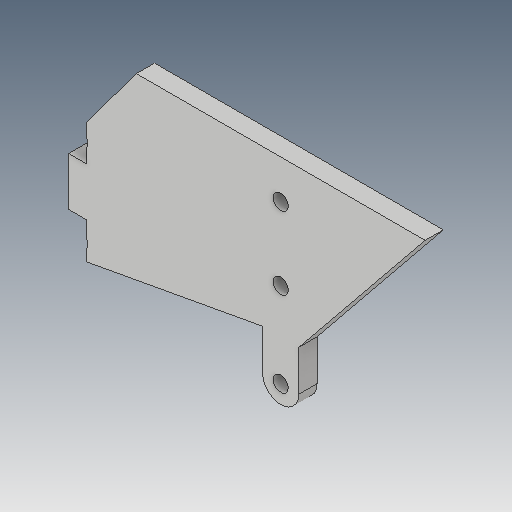
# Autodesk Inventor part: handPlate2
Saved by Autodesk Inventor 2019.4 (Build 234330000, 330)
## iProperties
Created: 2018-09-01
Part Number: handPlate2
Material: 一般
Document SubType Name: Modeling
Designer: AzLIer
Density: 1 g/cm^3
Appearance: 既定
Author: AzLIer
Autodesk Inventor part; units mm, degrees
ref_plane "YZ Plane" through (0, 0, 0) normal (1, 0, 0) x (0, 1, 0)
ref_plane "XZ Plane" through (0, 0, 0) normal (0, 1, 0) x (-1, 0, 0)
ref_plane "XY Plane" through (0, 0, 0) normal (0, 0, 1) x (1, 0, 0)
sketch "スケッチ1" plane through (0, 0, 0) normal (0, 0, 1) x (1, 0, 0)
  line L0 (0, 0) -> (-65, 0)
  line L1 (-65, 0) -> (-65, -60)
  line L2 (-65, -60) -> (0, -60)
  line L3 (0, -60) -> (0, 0)
  dimension "d0" = 65
  dimension "d1" = 60
  constraints: 8 end point, 2 parallel, 1 horizontal, 1 perpendicular
  measures "d0" distance of L2.end L1.end
  measures "d1" distance of L1.end L0.end
extrude "押し出し1" add sketch "スケッチ1" along normal blind 3
sketch "スケッチ2" plane through (0, 0, 3) normal (0, 0, 1) x (1, 0, 0)
  line L0 (-29, -25.6891) -> (-49.829, 0)
  line L1 (-2.171, 0) -> (-23, -25.6891)
  line L2 (-62, -31) -> (-65, -31)
  line L3 (-65, -31) -> (-65, -25)
  line L4 (-65, -25) -> (-62, -25)
  line L5 (-62, -25) -> (-62, -31)
  line L6 (-62, -17) -> (-65, -17)
  line L7 (-65, -17) -> (-65, -11)
  line L8 (-65, -11) -> (-62, -11)
  line L9 (-62, -11) -> (-62, -17)
  line L10 (-65, 4) -> (-62, 4)
  line L11 (-62, 4) -> (-62, 0)
  line L12 (-62, 0) -> (-65, 0)
  line L13 (-65, -4) -> (-65, 0)
  line L14 (-62, -4) -> (-65, -4)
  line L15 (-62, 0) -> (-62, -4)
  line L16 (-65, 0) -> (-65, 4)
  line L17 (-65, -40) -> (-62, -40)
  line L18 (0, 0) -> (0, -60) projected
  line L19 (0, -60) -> (-65, -60) projected
  line L20 (-65, -60) -> (-65, 0) projected
  line L21 (-65, 0) -> (0, 0) projected
  line L22 (-49.829, 0) -> (-62, -11)
  arc A0 (-29, -32.3891) -> (-23, -32.3891) centre (-26, -32.3891) ccw
  line L23 (-26, -32.3891) -> (-26, -29.3891) construction
  circle A1 centre (-26, -32.3891) radius 1.25
  line L24 (-23, -32.3891) -> (-23, -25.6891)
  line L25 (-29, -32.3891) -> (-29, -25.6891)
  circle A2 centre (-26, -18.3891) radius 1.25
  circle A3 centre (-26, -6.3891) radius 1.25
  line L26 (-29, -25.6891) -> (-62, -31)
  dimension "d4" = 6
  dimension "d5" = 2.5
  dimension "d6" = 3
  dimension "d7" = 2.5
  dimension "d8" = 2.5
  dimension "d9" = 14
  dimension "d10" = 26
  constraints: 46 end point, 10 vertical, 8 horizontal, 4 centre point, 4 point on line, 2 point on circle, 2 tangent, 1 coincident, 1 parallel, 20 other
  measures "d4" diameter of A0
  measures "d5" diameter of A1
  measures "d6" distance of L23.end L23.start
  measures "d7" diameter of A2
  measures "d8" diameter of A3
  measures "d9" distance of L23.start A2.centre
  measures "d10" distance of A3.centre L23.start
extrude "押し出し2" cut sketch "スケッチ2" against normal blind 3 contours L26 L5 L4 L20 L6 L9 L22 L0 | L0 L21 L1 L24 A0 L25 keep common part
sketch "スケッチ3" plane through (0, 0, 3) normal (0, 0, 1) x (1, 0, 0)
  circle A0 centre (-26, -6.3891) radius 1.25 projected
  circle A1 centre (-26, -18.3891) radius 1.25 projected
  circle A2 centre (-26, -32.3891) radius 1.25 projected
  line L0 (-62, -25) -> (-65, -25) projected
  line L1 (-65, -25) -> (-65, -17) projected
  line L2 (-65, -17) -> (-62, -17) projected
  line L3 (-62, -17) -> (-62, -11) projected
  line L4 (-62, -11) -> (-49.829, 0) projected
  line L5 (-49.829, 0) -> (-2.171, 0) projected
  line L6 (-2.171, 0) -> (-23, -25.6891) projected
  line L7 (-23, -25.6891) -> (-23, -32.3891) projected
  arc A3 (-29, -32.3891) -> (-23, -32.3891) centre (-26, -32.3891) ccw projected
  line L8 (-29, -32.3891) -> (-29, -25.6891) projected
  line L9 (-29, -25.6891) -> (-62, -31) projected
  line L10 (-62, -31) -> (-62, -25) projected
  arc A4 (-62, -28.9881) -> (-62, -27.7881) centre (-62.8, -28.3881) ccw
  arc A5 (-62, -14.6) -> (-62, -13.4) centre (-62.8, -14) ccw
  point P0 (0, 0)
  dimension "d13" = 2
  dimension "d14" = 2
  dimension "d15" = 3
  dimension "d16" = 3.3881
  dimension "d17" = 0.8
  constraints: 4 point on circle, 4 point on line, 2 centre point, 1 vertical alignment
  measures "d13" diameter of A4
  measures "d14" diameter of A5
  measures "d15" distance from line of L2 A5.centre
  measures "d16" distance from line of L0 A4.centre
  measures "d17" distance from line of L3 A5.centre
extrude "押し出し3" cut sketch "スケッチ3" against normal blind 3 contours A4 L10 | L3 A5
sketch "スケッチ4" plane through (0, 0, 3) normal (0, 0, 1) x (1, 0, 0)
  circle A0 centre (-26, -6.3891) radius 1.25 projected
  circle A1 centre (-26, -18.3891) radius 1.25 projected
  circle A2 centre (-26, -32.3891) radius 1.25 projected
  line L0 (-29, -32.3891) -> (-29, -25.6891) projected
  line L1 (-29, -25.6891) -> (-62, -31) projected
  line L2 (-62, -31) -> (-62, -28.9881) projected
  arc A3 (-62, -28.9881) -> (-62, -27.7881) centre (-62.8, -28.3881) ccw projected
  line L3 (-62, -27.7881) -> (-62, -25) projected
  line L4 (-62, -25) -> (-65, -25) projected
  line L5 (-65, -25) -> (-65, -17) projected
  line L6 (-65, -17) -> (-62, -17) projected
  line L7 (-62, -17) -> (-62, -14.6) projected
  arc A4 (-62, -14.6) -> (-62, -13.4) centre (-62.8, -14) ccw projected
  line L8 (-62, -13.4) -> (-62, -11) projected
  line L9 (-62, -11) -> (-49.829, 0) projected
  line L10 (-49.829, 0) -> (-2.171, 0) projected
  line L11 (-2.171, 0) -> (-23, -25.6891) projected
  line L12 (-23, -25.6891) -> (-23, -32.3891) projected
  arc A5 (-29, -32.3891) -> (-23, -32.3891) centre (-26, -32.3891) ccw projected
  line L13 (-58, -25) -> (-61, -25)
  line L14 (-61, -25) -> (-61, -17)
  line L15 (-61, -17) -> (-58, -17)
  line L16 (-65, -17) -> (-65, -25) projected
  line L17 (-62, -25) -> (-65, -25) projected
  circle A6 centre (-58.8, -28.3881) radius 1
  circle A7 centre (-58.8, -14) radius 1
  arc A8 (-62, -14.6) -> (-62, -13.4) centre (-62.8, -14) ccw projected
  line L18 (-49.829, 0) -> (-58, -11)
  line L19 (-58, -31) -> (-29, -25.6891)
  line L20 (-29, -25.6891) -> (-49.829, 0)
  line L21 (-58, -31) -> (-58, -28.9881)
  line L22 (-58, -27.7881) -> (-58, -25)
  line L23 (-58, -17) -> (-58, -14.6)
  line L24 (-58, -13.4) -> (-58, -11)
  dimension "d26" = 3
  dimension "d27" = 6
  dimension "d28" = 6
  dimension "d29" = 4
  constraints: 20 end point, 4 perpendicular, 4 point on circle, 2 centre point, 2 equal radius, 2 horizontal alignment, 2 vertical, 1 collinear, 1 parallel, 1 vertical alignment
  measures "d26" distance of L13.start L13.end
  measures "d27" distance of L19.start L13.start
  measures "d28" distance of L15.end L18.end
  measures "d29" distance between parallel lines of L5 L14
sketch "スケッチ5" plane through (0, 0, 3) normal (0, 0, 1) x (1, 0, 0)
  circle A0 centre (-26, -6.3891) radius 1.25 projected
  circle A1 centre (-26, -18.3891) radius 1.25 projected
  circle A2 centre (-26, -32.3891) radius 1.25 projected
  line L0 (-29, -32.3891) -> (-29, -25.6891) projected
  line L1 (-29, -25.6891) -> (-62, -31) projected
  line L2 (-62, -31) -> (-62, -28.9881) projected
  arc A3 (-62, -28.9881) -> (-62, -27.7881) centre (-62.8, -28.3881) ccw projected
  line L3 (-62, -27.7881) -> (-62, -25) projected
  line L4 (-62, -25) -> (-65, -25) projected
  line L5 (-65, -25) -> (-65, -17) projected
  line L6 (-65, -17) -> (-62, -17) projected
  line L7 (-62, -17) -> (-62, -14.6) projected
  arc A4 (-62, -14.6) -> (-62, -13.4) centre (-62.8, -14) ccw projected
  line L8 (-62, -13.4) -> (-62, -11) projected
  line L9 (-62, -11) -> (-49.829, 0) projected
  line L10 (-49.829, 0) -> (-2.171, 0) projected
  line L11 (-2.171, 0) -> (-23, -25.6891) projected
  line L12 (-23, -25.6891) -> (-23, -32.3891) projected
  arc A5 (-29, -32.3891) -> (-23, -32.3891) centre (-26, -32.3891) ccw projected
  circle A6 centre (-26, -6.3891) radius 1.25 projected
  circle A7 centre (-26, -18.3891) radius 1.25 projected
  circle A8 centre (-26, -32.3891) radius 1.25 projected
  line L13 (-29, -32.3891) -> (-29, -25.6891) projected
  line L14 (-29, -25.6891) -> (-62, -31) projected
  line L15 (-62, -31) -> (-62, -28.9881) projected
  arc A9 (-62, -28.9881) -> (-62, -27.7881) centre (-62.8, -28.3881) ccw projected
  line L16 (-62, -27.7881) -> (-62, -25) projected
  line L17 (-62, -25) -> (-65, -25) projected
  line L18 (-65, -25) -> (-65, -17) projected
  line L19 (-65, -17) -> (-62, -17) projected
  line L20 (-62, -17) -> (-62, -14.6) projected
  arc A10 (-62, -14.6) -> (-62, -13.4) centre (-62.8, -14) ccw projected
  line L21 (-62, -13.4) -> (-62, -11) projected
  line L22 (-62, -11) -> (-49.829, 0) projected
  line L23 (-49.829, 0) -> (-2.171, 0) projected
  line L24 (-2.171, 0) -> (-23, -25.6891) projected
  line L25 (-23, -25.6891) -> (-23, -32.3891) projected
  arc A11 (-29, -32.3891) -> (-23, -32.3891) centre (-26, -32.3891) ccw projected
  circle A12 centre (-26, -6.3891) radius 1.25 projected
  circle A13 centre (-26, -18.3891) radius 1.25 projected
  circle A14 centre (-26, -32.3891) radius 1.25 projected
  line L26 (-29, -32.3891) -> (-29, -25.6891) projected
  line L27 (-29, -25.6891) -> (-62, -31) projected
  line L28 (-62, -31) -> (-62, -28.9881) projected
  arc A15 (-62, -28.9881) -> (-62, -27.7881) centre (-62.8, -28.3881) ccw projected
  line L29 (-62, -27.7881) -> (-62, -25) projected
  line L30 (-62, -25) -> (-65, -25) projected
  line L31 (-65, -25) -> (-65, -17) projected
  line L32 (-65, -17) -> (-62, -17) projected
  line L33 (-62, -17) -> (-62, -14.6) projected
  arc A16 (-62, -14.6) -> (-62, -13.4) centre (-62.8, -14) ccw projected
  line L34 (-62, -13.4) -> (-62, -11) projected
  line L35 (-62, -11) -> (-49.829, 0) projected
  line L36 (-49.829, 0) -> (-2.171, 0) projected
  line L37 (-2.171, 0) -> (-23, -25.6891) projected
  line L38 (-23, -25.6891) -> (-23, -32.3891) projected
  arc A17 (-29, -32.3891) -> (-23, -32.3891) centre (-26, -32.3891) ccw projected
  arc A18 (-62, -14.6) -> (-62, -13.4) centre (-62.8, -14) ccw projected
  line L39 (-62, -17) -> (-62, -14.6) projected
  line L40 (-65, -17) -> (-62, -17) projected
  line L41 (-65, -17) -> (-65, -25) projected
  line L42 (-62, -25) -> (-65, -25) projected
  line L43 (-62, -27.7881) -> (-62, -25) projected
  arc A19 (-62, -28.9881) -> (-62, -27.7881) centre (-62.8, -28.3881) ccw projected
  line L44 (-62, -31) -> (-62, -28.9881) projected
  line L45 (-29, -25.6891) -> (-62, -31) projected
  line L46 (-29, -32.3891) -> (-29, -25.6891) projected
  arc A20 (-29, -32.3891) -> (-23, -32.3891) centre (-26, -32.3891) ccw projected
  line L47 (-23, -25.6891) -> (-23, -32.3891) projected
  line L48 (-2.171, 0) -> (-23, -25.6891) projected
  line L49 (-2.171, 0) -> (-49.829, 0) projected
  line L50 (-62, -11) -> (-49.829, 0) projected
  line L51 (-62, -13.4) -> (-62, -11) projected
  circle A21 centre (-26, -32.3891) radius 1.25 projected
  circle A22 centre (-26, -18.3891) radius 1.25 projected
  circle A23 centre (-26, -6.3891) radius 1.25 projected
  line L52 (-29, -25.6891) -> (-49.829, 0)
  line L53 (-29, -25.6891) -> (-65.9346, -36.6422)
  line L54 (-65.9346, -36.6422) -> (-73.9425, -10.887)
  line L55 (-73.9425, -10.887) -> (-49.829, 0)
  point P0 (0, 0)
  constraints: 8 end point
extrude "押し出し4" cut sketch "スケッチ5" against normal blind 3 contours L1 L2 A3 L3 L4 L5 L6 L7 A4 L8 L9 L52
extrude "押し出し5" add sketch "スケッチ4" against normal blind 3 contours L19 L21 L1 | L1 L21 A6 L22 L13 L14 L15 L23 A7 L24 L18 L20
equation "\"d28\" = d27"
